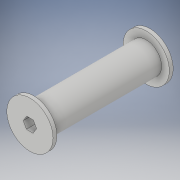
# Autodesk Inventor part: Polycord conveyor
Saved by Autodesk Inventor 2018 (Build 220112000, 112)
## iProperties
Created: 2020-01-29
Part Number: Polycord conveyor
Material: Generic
Document SubType Name: Modeling
Designer: s-4008082
Density: 1 g/cm^3
Appearance: Default
Author: s-4008082
Autodesk Inventor part; units mm, degrees
ref_plane "YZ Plane" through (0, 0, 0) normal (1, 0, 0) x (0, 1, 0)
ref_plane "XZ Plane" through (0, 0, 0) normal (0, 1, 0) x (-1, 0, 0)
ref_plane "XY Plane" through (0, 0, 0) normal (0, 0, 1) x (1, 0, 0)
sketch "Sketch1" plane through (0, 0, 0) normal (0, 0, 1) x (1, 0, 0)
  line L0 (-5.4972, 0.152) -> (-2.6169, 4.8367)
  line L1 (-2.6169, 4.8367) -> (2.8802, 4.6847)
  line L2 (2.8802, 4.6847) -> (5.4972, -0.152)
  line L3 (5.4972, -0.152) -> (2.6169, -4.8367)
  line L4 (2.6169, -4.8367) -> (-2.8802, -4.6847)
  line L5 (-2.8802, -4.6847) -> (-5.4972, 0.152)
  circle A0 centre (0, 0) radius 12.7
  dimension "d0" = 9.525
  dimension "d1" = 25.4
  constraints: 12 end point, 2 coincident, 1 centre point, 13 other
  measures "d0" distance between parallel lines of L4 L1
  measures "d1" diameter of A0
extrude "Extrusion1" add sketch "Sketch1" along normal blind 92.71
sketch "Sketch3" plane through (0, 0, 92.71) normal (0, 0, 1) x (1, 0, 0)
  line L0 (-5.4972, 0.152) -> (-2.6169, 4.8367) projected
  line L1 (-5.4972, 0.152) -> (-2.6169, 4.8367)
  line L2 (-2.6169, 4.8367) -> (2.8802, 4.6847)
  line L3 (2.8802, 4.6847) -> (5.4972, -0.152)
  line L4 (5.4972, -0.152) -> (2.6169, -4.8367)
  line L5 (2.6169, -4.8367) -> (-2.8802, -4.6847)
  line L6 (-2.8802, -4.6847) -> (-5.4972, 0.152)
  circle A0 centre (0, 0) radius 19.05
  dimension "d4" = 38.1
  constraints: 12 end point, 2 coincident, 1 centre point, 13 other
  measures "d4" diameter of A0
extrude "Extrusion2" add sketch "Sketch3" along normal blind 3.175
sketch "Sketch4" plane through (0, 0, 0) normal (0, 0, -1) x (-1, 0, 0)
  line L0 (-7.3295, -0.2027) -> (-3.8403, 6.2462)
  line L1 (-3.8403, 6.2462) -> (3.4893, 6.4489)
  line L2 (3.4893, 6.4489) -> (7.3295, 0.2027)
  line L3 (7.3295, 0.2027) -> (3.8403, -6.2462)
  line L4 (3.8403, -6.2462) -> (-3.4893, -6.4489)
  line L5 (-3.4893, -6.4489) -> (-7.3295, -0.2027)
  line L6 (2.8802, -4.6847) -> (-2.6169, -4.8367) projected
  circle A0 centre (0, 0) radius 19.05
  dimension "d7" = 12.7
  dimension "d8" = 180
  dimension "d11" = 38.1
  constraints: 12 end point, 2 coincident, 1 centre point, 13 other
  measures "d7" distance between parallel lines of L4 L1
  measures "d8" angle of L6 L4
  measures "d11" diameter of A0
extrude "Extrusion3" add sketch "Sketch4" along normal blind 3.175
body "Solid1"
